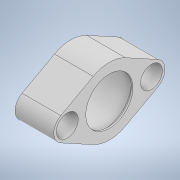
# Autodesk Inventor part: XY Drive Bearing Holder
Saved by Autodesk Inventor 2022 (Build 260153000, 153)
## iProperties
Created: 2021-10-05
Part Number: XY Drive Bearing Holder
Material: Generic
Document SubType Name: Modeling
Designer: Administrator
Density: 1 g/cm^3
Appearance: Default
Mass: 2.31591 g
Surface Area: 23.5459 cm^2
Volume: 2.31591 cm^3
Title: XY Drive Bearing Holder v9
Author: Administrator
Autodesk Inventor part; units mm, degrees
ref_plane "XZ Plane" through (0, 0, 0) normal (0, 1, 0) x (-1, 0, 0)
ref_plane "XY Plane" through (0, 0, 0) normal (0, 0, 1) x (1, 0, 0)
ref_plane "Work Plane1" through (-10, 0, 0) normal (1, 0, 0) x (0, 1, 0)
sketch "Sketch1" plane through (-10, 0, 0) normal (1, 0, 0) x (0, 1, 0)
  line L0 (3.5091, 14.42) -> (8.7727, 4.8)
  arc A0 (-8.7727, 4.8) -> (-8.7727, -4.8) centre (0, 0) ccw
  line L1 (8.7727, -4.8) -> (3.5091, -14.42)
  arc A1 (3.5091, 14.42) -> (-3.5091, 14.42) centre (0, 12.5) ccw
  line L2 (-3.5091, -14.42) -> (-8.7727, -4.8)
  arc A2 (8.7727, -4.8) -> (8.7727, 4.8) centre (0, 0) ccw
  line L3 (-8.7727, 4.8) -> (-3.5091, 14.42)
  arc A3 (-3.5091, -14.42) -> (3.5091, -14.42) centre (0, -12.5) ccw
  constraints: 8 end point, 8 point on circle, 4 centre point, 3 equal length, 2 parallel
extrude "Extrusion1" add sketch "Sketch1" along normal blind 11.5
hole "Hole4" at (1.5, 0, 0) direction (-1, 0, 0) diameter 14 depth 11.5 tip angle 118
hole "Hole3" at (1.5, 0, -12.5) direction (-1, 0, 0) diameter 3.2 depth 11.5 counterbore diameter 6.5 counterbore depth 6
sketch "Sketch3" plane through (1.5, 0, 0) normal (1, 0, 0) x (0, 0, -1)
  point P0 (12.5, 0)
hole "Hole2" at (1.5, 0, 12.5) direction (-1, 0, 0) diameter 3.2 depth 11.5 counterbore diameter 6.5 counterbore depth 6
sketch "Sketch2" plane through (1.5, 0, 0) normal (1, 0, 0) x (0, 0, -1)
  point P0 (0, 0)
hole "Hole1" at (-10, 0, 0) direction (1, 0, 0) diameter 16 depth 10 tip angle 90
chamfer "Chamfer3" distance 0.5 angle 45 1 edges at (-10, 0, -10.9)
chamfer "Chamfer2" distance 0.5 angle 45 1 edges at (-10, 0, 14.1)
chamfer "Chamfer1" distance 0.5 angle 45 1 edges at (-10, 0, -8)
sketch "Sketch4" plane through (1.5, 0, 0) normal (1, 0, 0) x (0, 0, -1)
  point P0 (-12.5, 0)
sketch "Sketch5" plane through (-10, 0, 0) normal (1, 0, 0) x (0, 1, 0)
  point P0 (0, 0)
body "Solid3"
